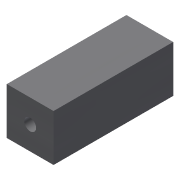
# Autodesk Inventor part: parameters
Saved by Autodesk Inventor 2022 Beta2 (Build 260130000, 130) ContinuousBuild 0
## iProperties
Shininess: 64.0
Length Units: 11269
Angle Units: 11279
Time Units: 11290
Mass Units: 11283
Length Display Precision: 3
Angle Display Precision: 2
Created: 2002-04-17
Part Number: parameters
Document SubType Name: Modeling
Designer: Administrator
Density: 1 g/cm^3
Material: Generic
Appearance: Light Gray
Density: 0.0
Volumn: 0.0
Area: 0.0
PropertySet Name: Model Information
Control State: 0
Master: False
Checked Out: False
Author: Administrator
Autodesk Inventor part; units mm, degrees
ref_plane "YZ Plane" through (0, 0, 0) normal (1, 0, 0) x (0, 1, 0)
ref_plane "XZ Plane" through (0, 0, 0) normal (0, 1, 0) x (-1, 0, 0)
ref_plane "XY Plane" through (0, 0, 0) normal (0, 0, 1) x (1, 0, 0)
sketch "Sketch1" plane through (0, 0, 0) normal (0, 0, 1) x (1, 0, 0)
  line L0 (-21.5328, 23.6618) -> (3.4672, 23.6618)
  line L1 (3.4672, 23.6618) -> (3.4672, -1.3382)
  line L2 (3.4672, -1.3382) -> (-21.5328, -1.3382)
  line L3 (-21.5328, -1.3382) -> (-21.5328, 23.6618)
  dimension "d0" = 25
  dimension "d1" = 25
  constraints: 8 end point, 2 parallel, 1 horizontal, 1 perpendicular
  measures "d0" distance of L1.end L2.end
  measures "d1" distance of L2.end L0.start
extrude "Extrusion1" add sketch "Sketch1" along normal blind 64
sketch "Sketch2" plane through (0, 0, 64) normal (0, 0, 1) x (1, 0, 0)
  line L0 (3.4672, 23.6618) -> (3.4672, -1.3382) projected
  line L1 (-21.5328, 23.6618) -> (3.4672, 23.6618) projected
  line L2 (-21.5328, -1.3382) -> (-21.5328, 23.6618) projected
  circle A0 centre (-9.0328, 11.1618) radius 12.5 construction
  constraints: 3 tangent, 2 coincident, 1 centre point
hole "Hole1" at (-9.0328, 11.1618, 64) at (-9.0328, 11.1618, 64) direction (0, 0, -1) diameter 6.35 end through all
body "Solid1"
